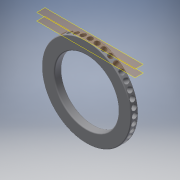
# Autodesk Inventor part: InnerRingAJB
Saved by Autodesk Inventor 2018 (Build 220112000, 112)
## iProperties
Created: 2018-02-16
Part Number: InnerRingAJB
Material: Generic
Document SubType Name: Modeling
Designer: Alec temporary
Density: 1 g/cm^3
Appearance: Default
Author: Alec temporary
Autodesk Inventor part; units mm, degrees
ref_plane "YZ Plane" through (0, 0, 0) normal (1, 0, 0) x (0, 1, 0)
ref_plane "XY Plane" through (0, 0, 0) normal (0, 0, 1) x (1, 0, 0)
sketch "Sketch1" plane through (0, 0, 0) normal (0, 0, 1) x (1, 0, 0)
  spline S0 degree 3 number of poles 66 construction
  spline S1 degree 3 number of poles 66 construction
  spline S2 degree 3 number of poles 66 construction
  spline S3 degree 3 number of poles 66 construction
  line L0 (0, 0) -> (-1289.5077, 1289.5077) construction
  line L1 (0, 0) -> (-1733.0494, 0) construction
  line L2 (-1054.526, 1524.4998) -> (-1432.5934, 1146.4324) construction
  line L3 (0, 0) -> (878.1604, 878.1604) construction
  spline S4 degree 3 number of poles 66 construction
  line L4 (1382.491, 1196.5349) -> (1052.4766, 1526.5492) construction
  line L5 (0, 0) -> (-741.9195, -741.9195) construction
  spline S5 degree 3 number of poles 66 construction
  line L6 (-1102.1411, -1491.4606) -> (-1490.5364, -1103.0653) construction
  circle A0 centre (0, -7.2879) radius 1828.8 construction
  circle A1 centre (0, -7.2879) radius 1524.0029
  line L7 (1523.9855, 0) -> (1828.7855, 0) construction
  circle A2 centre (0, -7.2879) radius 2133.5979
  line L8 (1828.7855, 0) -> (2133.5855, 0) construction
  point P0 (1401.5066, 1167.5694)
  point P1 (-1174.8573, 1394.2186)
  point P2 (-1683.0762, 708.0895)
  point P3 (1200.4635, 1372.3488)
  point P4 (-1200.4635, -1386.9247)
  dimension "d0" = 45
  dimension "d1" = 135
  dimension "d2" = 45
  dimension "d3" = 304.8
  dimension "d4" = 304.8
  constraints: 18 end point, 3 horizontal, 3 perpendicular, 2 coincident, 1 collinear, 16 other
  measures "d0" angle of L0 L1
  measures "d1" angle of L1 L3
  measures "d2" angle of L1 L5
  measures "d3" distance of L7.start L7.end
  measures "d4" distance of L7.end L8.end
extrude "Extrusion1" add sketch "Sketch1" along normal mid plane 355.6
ref_plane "Work Plane2" through (0, 1770.71, 0) normal (0, 1, 0) x (-1, 0, 0)
ref_plane "Work Plane1" through (0, 2126.31, 0) normal (0, 1, 0) x (-1, 0, 0)
sketch "Sketch2" plane through (0, 1770.71, 0) normal (0, 1, 0) x (-1, 0, 0)
  circle A0 centre (-7.2879, 0) radius 127 projected
  point P0 (0, 0)
extrude "Extrusion2" cut sketch "Sketch2" along normal blind 355.6
pattern_circular "Circular Pattern1" count 40 over 360 about axis through (0, -7.2879, 0) along (0, 0, 1) of "Extrusion2"
chamfer "Chamfer1" distance 25.4 angle 45 2 edges at (-2133.5979, -7.2879, -177.8) (-2133.5979, -7.2879, 177.8)
fillet "Fillet1" radius 25.4 4 edges at (-2133.5979, -7.2879, 152.4) (-2108.1979, -7.2879, 177.8) (-2133.5979, -7.2879, -152.4) (-2108.1979, -7.2879, -177.8)
fillet "Fillet2" radius 50.8 2 edges at (-1524.0029, -7.2879, -177.8) (-1524.0029, -7.2879, 177.8)
body "Solid1"
